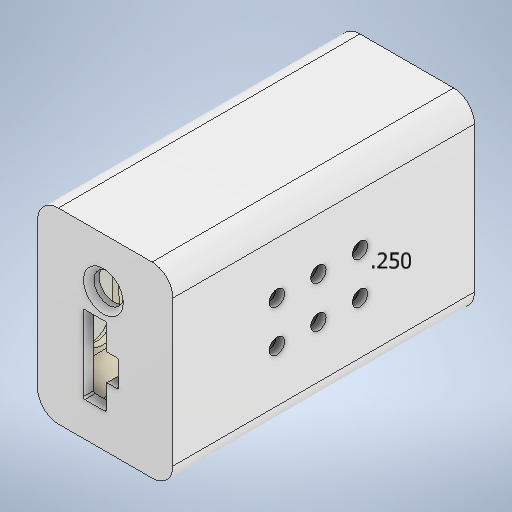
# Autodesk Inventor part: Battery Holder
Saved by Autodesk Inventor 2025.1 (Build 291241020, 241B)
## iProperties
Created: 2024-12-04
Part Number: Battery Holder
Material: ABS Plastic
Document SubType Name: Modeling
Designer: AtuStem
Mass: 53.2427 g
Surface Area: 327.859 cm^2
Volume: 53.2427 cm^3
Density: 1.06 g/cm^3
Appearance: Smooth - White
Author: AtuStem
Autodesk Inventor part; units mm, degrees
ref_plane "YZ Plane" through (0, 0, 0) normal (1, 0, 0) x (0, 1, 0)
ref_plane "XZ Plane" through (0, 0, 0) normal (0, 1, 0) x (-1, 0, 0)
ref_plane "XY Plane" through (0, 0, 0) normal (0, 0, 1) x (1, 0, 0)
ref_plane "Work Plane1" through (0, 0, 0) normal (0, 0, 1) x (1, 0, 0)
sketch "Sketch1" plane through (0, 0, 0) normal (0, 0, 1) x (1, 0, 0)
  line L0 (-18.547, -42.0159) -> (5.3123, -42.6404)
  line L1 (5.3123, -42.6404) -> (5.3123, -3.8596)
  line L2 (5.3123, -3.8596) -> (-18.547, -4.4841)
  spline S0 degree 2 poles (-18.547, -4.4841) (-18.5491, -23.25) (-18.547, -42.0159) knots 0 0 0 1 1 1
  line L3 (-9.1323, -33.49) -> (-6.2213, -33.49)
  ellipse E0 centre (-9.1323, -33.59) end of major axis (-9.2323, -33.59) minor radius 0.1 (-9.1323, -33.49) -> (-9.2323, -33.59) ccw
  line L4 (-9.2323, -40.82) -> (-9.2323, -33.59)
  ellipse E1 centre (-9.7325, -40.82) end of major axis (-10.2326, -40.82) minor radius 0.5 (-9.7325, -41.32) -> (-9.2323, -40.82) ccw
  line L5 (-15.8746, -41.32) -> (-9.7325, -41.32)
  ellipse E2 centre (-15.8746, -40.82) end of major axis (-16.3747, -40.82) minor radius 0.5 (-16.3747, -40.82) -> (-15.8746, -41.32) ccw
  line L6 (-16.3747, -18.02) -> (-16.3747, -40.82)
  ellipse E3 centre (-15.8746, -18.02) end of major axis (-16.3747, -18.02) minor radius 0.5 (-15.8746, -17.52) -> (-16.3747, -18.02) ccw
  line L7 (-9.7325, -17.52) -> (-15.8746, -17.52)
  ellipse E4 centre (-9.7325, -18.02) end of major axis (-10.2326, -18.02) minor radius 0.5 (-9.2323, -18.02) -> (-9.7325, -17.52) ccw
  line L8 (-9.2323, -25.25) -> (-9.2323, -18.02)
  ellipse E5 centre (-9.1323, -25.25) end of major axis (-9.2323, -25.25) minor radius 0.1 (-9.2323, -25.25) -> (-9.1323, -25.35) ccw
  line L9 (-6.2213, -25.35) -> (-9.1323, -25.35)
  ellipse E6 centre (-6.2213, -26.1) end of major axis (-6.9715, -26.1) minor radius 0.75 (-5.471, -26.1) -> (-6.2213, -25.35) ccw
  line L10 (-5.471, -32.74) -> (-5.471, -26.1)
  ellipse E7 centre (-6.2213, -32.74) end of major axis (-6.9715, -32.74) minor radius 0.75 (-6.2213, -33.49) -> (-5.471, -32.74) ccw
  line L11 (-3.1011, -5.2) -> (-14.2049, -5.2)
  ellipse E8 centre (-3.1011, -5.3) end of major axis (-3.2011, -5.3) minor radius 0.1 (-3.001, -5.3) -> (-3.1011, -5.2) ccw
  line L12 (-3.001, -14.4) -> (-3.001, -5.3)
  ellipse E9 centre (-3.1011, -14.4) end of major axis (-3.2011, -14.4) minor radius 0.1 (-3.1011, -14.5) -> (-3.001, -14.4) ccw
  line L13 (-14.2049, -14.5) -> (-3.1011, -14.5)
  ellipse E10 centre (-14.2049, -14.4) end of major axis (-14.3049, -14.4) minor radius 0.1 (-14.3049, -14.4) -> (-14.2049, -14.5) ccw
  line L14 (-14.3049, -5.3) -> (-14.3049, -14.4)
  ellipse E11 centre (-14.2049, -5.3) end of major axis (-14.3049, -5.3) minor radius 0.1 (-14.2049, -5.2) -> (-14.3049, -5.3) ccw
  line L15 (-3.1594, -14.35) -> (-14.1556, -14.35)
  line L16 (-3.1594, -14.35) -> (-3.1594, -5.35)
  line L17 (-14.1556, -5.35) -> (-3.1594, -5.35)
  line L18 (-14.1556, -5.35) -> (-14.1556, -14.35)
  ellipse E12 centre (-10.1978, -9.85) end of major axis (-10.1978, -6.6) minor radius 3.2489
  circle A0 centre (-10.1978, -9.85) radius 4.445
  point P0 (0, 0)
  point P1 (-18.548, -23.25)
  dimension "d3" = 8.89
  dimension "d56" = 10.7833
  dimension "d57" = 15.5101
  constraints: 38 end point, 1 centre point, 1 vertical, 54 other
  measures "d3" diameter of A0
  measures "d56" distance between parallel lines of L1 L10
  measures "d57" distance from line of L1 A0.centre
extrude "Extrusion2" add sketch "Sketch1" along normal blind 3.175 contours S0 L2 L1 L0 | E8 L12 E9 L13 E10 L14 A0 L18 L15 L16 L17 E11 L11 | L18 L17 L16 L15 A0
sketch "Sketch2" plane through (0, 0, 0) normal (0, 0, 1) x (1, 0, 0)
  line L0 (-24.9349, -6.9281) -> (-22.8012, -6.9281) projected
  line L1 (7.5493, -6.5903) -> (5.6096, -6.5903) projected
  line L2 (-1.1057, -0.0262) -> (3.5072, -0.147) projected
  line L3 (3.5072, -46.353) -> (-1.1057, -46.4738) projected
  line L4 (-25.1889, -46.7278) -> (5.9261, -46.7278) construction
  line L5 (5.9261, -46.7278) -> (5.9261, 0.2278) construction
  line L6 (5.9261, 0.2278) -> (-25.1889, 0.2278) construction
  line L7 (-25.1889, 0.2278) -> (-25.1889, -46.7278) construction
  line L8 (-25.1889, -46.7278) -> (5.9261, -46.7278)
  line L9 (5.9261, -46.7278) -> (5.9261, 0.2278)
  line L10 (5.9261, 0.2278) -> (-25.1889, 0.2278)
  line L11 (-25.1889, 0.2278) -> (-25.1889, -46.7278)
  line L12 (-30.2689, -51.8078) -> (11.0061, -51.8078)
  line L13 (11.0061, -51.8078) -> (11.0061, 5.3078)
  line L14 (11.0061, 5.3078) -> (-30.2689, 5.3078)
  line L15 (-30.2689, 5.3078) -> (-30.2689, -51.8078)
  point P0 (0, 0)
  dimension "d6" = 0
  dimension "d7" = 5.08
  dimension "d55" = 31.115
  constraints: 24 end point, 6 parallel, 3 perpendicular, 1 horizontal, 6 other
  measures "d6" distance between parallel lines of L7 L11
  measures "d7" distance between parallel lines of L11 L15
  measures "d55" distance between parallel lines of L5 L11
extrude "Extrusion3" add sketch "Sketch2" against normal blind 88.9
sketch "Sketch3" plane through (0, 0, 0) normal (0, 0, 1) x (1, 0, 0)
  line L0 (11.0061, 5.3078) -> (-30.2689, 5.3078) projected
  line L1 (-30.2689, 5.3078) -> (-30.2689, -51.8078) projected
  line L2 (11.0061, -51.8078) -> (11.0061, 5.3078) projected
  line L3 (-30.2689, -51.8078) -> (11.0061, -51.8078) projected
  line L4 (5.3123, -42.6404) -> (5.3123, -3.8596) projected
  line L5 (5.3123, -3.8596) -> (-18.547, -4.4841) projected
  spline S0 degree 2 poles (-18.547, -4.4841) (-18.5491, -23.25) (-18.547, -42.0159) knots 0 0 0 1 1 1 projected
  line L6 (-18.547, -42.0159) -> (5.3123, -42.6404) projected
  ellipse E0 centre (-9.1323, -25.25) end of major axis (-9.2323, -25.25) minor radius 0.1 (-9.2323, -25.25) -> (-9.1323, -25.35) ccw projected
  line L7 (-9.1323, -25.35) -> (-6.2213, -25.35) projected
  ellipse E1 centre (-6.2213, -26.1) end of major axis (-5.471, -26.1) minor radius 0.75 (-5.471, -26.1) -> (-6.2213, -25.35) ccw projected
  line L8 (-5.471, -26.1) -> (-5.471, -32.74) projected
  ellipse E2 centre (-6.2213, -32.74) end of major axis (-5.471, -32.74) minor radius 0.75 (-6.2213, -33.49) -> (-5.471, -32.74) ccw projected
  line L9 (-6.2213, -33.49) -> (-9.1323, -33.49) projected
  ellipse E3 centre (-9.1323, -33.59) end of major axis (-9.2323, -33.59) minor radius 0.1 (-9.1323, -33.49) -> (-9.2323, -33.59) ccw projected
  line L10 (-9.2323, -33.59) -> (-9.2323, -40.82) projected
  ellipse E4 centre (-9.7325, -40.82) end of major axis (-9.2323, -40.82) minor radius 0.5 (-9.7325, -41.32) -> (-9.2323, -40.82) ccw projected
  line L11 (-9.7325, -41.32) -> (-15.8746, -41.32) projected
  ellipse E5 centre (-15.8746, -40.82) end of major axis (-15.3744, -40.82) minor radius 0.5 (-16.3747, -40.82) -> (-15.8746, -41.32) ccw projected
  line L12 (-16.3747, -40.82) -> (-16.3747, -18.02) projected
  ellipse E6 centre (-15.8746, -18.02) end of major axis (-15.3744, -18.02) minor radius 0.5 (-15.8746, -17.52) -> (-16.3747, -18.02) ccw projected
  line L13 (-15.8746, -17.52) -> (-9.7325, -17.52) projected
  ellipse E7 centre (-9.7325, -18.02) end of major axis (-9.2323, -18.02) minor radius 0.5 (-9.2323, -18.02) -> (-9.7325, -17.52) ccw projected
  line L14 (-9.2323, -18.02) -> (-9.2323, -25.25) projected
  circle A0 centre (-10.1978, -9.85) radius 4.445 projected
  point P0 (0, 0)
  constraints: 1 vertical alignment, 8 other
extrude "Extrusion4" add sketch "Sketch3" along normal blind 3.175 contours L2 L3 L1 L0
sketch "Sketch4" plane through (-30.2689, -51.8078, -88.9) normal (-1, 0, 0) x (0, 0, 1)
  ellipse E0 centre (77.4131, 34.4328) end of major axis (77.4131, 32.3872) minor radius 2.045 (78.4721, 32.6828) -> (76.3541, 32.6828) ccw projected
  ellipse E1 centre (77.3843, 17.9328) end of major axis (77.3843, 13.6828) minor radius 4.2485 (75.9017, 21.9156) -> (76.7687, 13.7277) ccw projected
  circle A0 centre (77.4131, 34.4328) radius 5.08
  circle A1 centre (77.3843, 17.9328) radius 5.08
  line L0 (72.3043, 17.9417) -> (72.3331, 34.4417)
  line L1 (82.4931, 34.424) -> (82.4643, 17.924)
  point P0 (88.9, 51.8078)
  point P1 (82.4643, 16.0278)
  point P2 (82.4643, 19.2028)
  point P3 (82.4643, 17.9328)
  dimension "d15" = 10.16
  dimension "d16" = 10.16
  constraints: 4 end point, 4 point on circle, 4 tangent, 2 centre point, 2 coincident, 2 other
  measures "d15" diameter of A0
  measures "d16" diameter of A1
extrude "Extrusion5" cut sketch "Sketch4" against normal up to next
chamfer "Chamfer1" distance 3.175 angle 45 4 edges at (-30.2689, -38.955, -11.5201) (-30.2689, -25.6161, -16.5813) (-30.2689, -12.295, -11.478) (-30.2689, -25.6294, -6.4213)
chamfer "Chamfer2" distance 1.5875 angle 45 1 edges at (-14.6428, -9.85, 3.175)
fillet "Fillet1" radius 6.35 4 edges at (-30.2689, 5.3078, -42.8625) (-30.2689, -51.8078, -42.8625) (11.0061, -51.8078, -42.8625) (11.0061, 5.3078, -42.8625)
fillet "Fillet2" radius 6.35 4 edges at (-25.1889, 0.2278, -44.45) (5.9261, 0.2278, -44.45) (5.9261, -46.7278, -44.45) (-25.1889, -46.7278, -44.45)
sketch "Sketch5" plane through (5.9261, -40.3778, 0) normal (-1, 0, 0) x (0, 0, 1)
  arc A0 (-19.7707, 6.5172) -> (-3.2607, 6.5028) centre (-11.5157, 6.5028) ccw projected
  line L0 (-19.7419, 23.0172) -> (-19.7707, 6.5172) projected
  arc A1 (-3.2319, 22.9884) -> (-19.7419, 23.0172) centre (-11.4869, 23.0028) ccw projected
  line L1 (-3.2607, 6.5028) -> (-3.2319, 22.9884) projected
  line L2 (3.175, -5.08) -> (-88.9, -5.08) projected
  line L3 (3.175, 39.3357) -> (3.175, -5.08) projected
  line L4 (-88.9, 39.3357) -> (3.175, 39.3357) projected
  line L5 (-88.9, -5.08) -> (-88.9, 39.3357) projected
  line L6 (-88.9, 39.3357) -> (-88.9, 45.6857) projected
  line L7 (-88.9, 39.3357) -> (-69.85, 39.3357)
  line L8 (-88.9, -5.08) -> (3.175, -5.08) projected
  line L9 (3.175, -5.08) -> (-28.575, -5.08)
  line L10 (-28.575, -5.08) -> (-28.575, 39.3357)
  line L11 (-28.575, 17.1278) -> (-28.575, 21.5728)
  line L12 (-28.575, 17.1278) -> (-28.575, 10.7778)
  point P0 (0, 40.3778)
  dimension "d28" = 31.75
  dimension "d31" = 6.35
  constraints: 10 end point, 5 point on line, 1 coincident, 1 midpoint, 1 perpendicular
  measures "d28" distance of L2.start L9.end
  measures "d31" distance of L11.start L12.end
hole "Hole1" at (5.9261, -29.6, -28.575) direction (1, 0, 0) diameter 4.6482 end through all counterbore diameter 8.255 counterbore depth 2.54
pattern_linear "Rectangular Pattern1" count 2 spacing 12.7 along (0, 1, 0) count 3 spacing 12.7 along (0, 0, -1) of "Hole1"
sketch "Sketch6" plane through (5.9261, -40.3778, 0) normal (-1, 0, 0) x (0, 0, 1)
  circle A0 centre (-28.575, 23.4778) radius 2.3241 projected
  circle A1 centre (-28.575, 10.7778) radius 2.3241 projected
  circle A2 centre (-41.275, 10.7778) radius 2.3241 projected
  circle A3 centre (-41.275, 23.4778) radius 2.3241 projected
  circle A4 centre (-53.975, 23.4778) radius 2.3241 projected
  circle A5 centre (-53.975, 10.7778) radius 2.3241 projected
  point P0 (0, 40.3778)
sketch "Sketch7" plane through (-18.8389, -46.7278, 0) normal (0, 1, 0) x (1, 0, 0)
  line L0 (-5.08, 88.9) -> (23.495, 88.9) projected
  line L1 (9.2075, 88.9) -> (9.2075, 82.55)
  point P0 (18.8389, 0)
  dimension "d45" = 6.35
  constraints: 2 end point, 1 coincident, 1 midpoint, 1 vertical
  measures "d45" distance of L1.start L1.end
extrude "Extrusion6" cut sketch "Sketch6" along normal up to next
body "Solid2"
